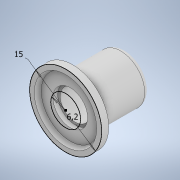
# Autodesk Inventor part: KnopfDuenn
Saved by Autodesk Inventor 2022.2 (Build 262287010, 287A)
## iProperties
Created: 2022-01-27
Part Number: KnopfDuenn
Material: Generisch
Document SubType Name: Modeling
Designer: hpcwoess
Density: 1 g/cm^3
Appearance: Vorgabe
Author: hpcwoess
Autodesk Inventor part; units mm, degrees
ref_plane "YZ Plane" through (0, 0, 0) normal (1, 0, 0) x (0, 1, 0)
ref_plane "XZ Plane" through (0, 0, 0) normal (0, 1, 0) x (-1, 0, 0)
ref_plane "XY Plane" through (0, 0, 0) normal (0, 0, 1) x (1, 0, 0)
sketch "Skizze1" plane through (0, 0, 0) normal (0, 0, 1) x (1, 0, 0)
  circle A0 centre (0, 0) radius 3.1
  circle A1 centre (0, 0) radius 7.5
  dimension "d0" = 6.2
  dimension "d1" = 15
  constraints: 2 centre point, 2 coincident
  measures "d0" diameter of A0
  measures "d1" diameter of A1
sketch "Skizze2" plane through (0, 0, 0) normal (1, 0, 0) x (0, 1, 0)
  line L0 (3.1, -2) -> (3.1, -11.5)
  line L1 (3.1, -11.5) -> (0, -11.5)
  line L2 (0, -11.5) -> (0, -12.5)
  line L3 (0, -12.5) -> (5, -12.5)
  line L4 (5, -12.5) -> (5, -2.5)
  line L5 (5, -2.5) -> (7.5, -1.5)
  line L6 (7.5, -1.5) -> (7.5, 0)
  line L7 (7.5, 0) -> (6.5, 0)
  line L8 (-10.5, 0) -> (10.5, 0) projected
  line L9 (0, -15) -> (0, 2.5) projected
  line L10 (3.6, -1) -> (3.6, -2)
  line L11 (3.6, -2) -> (3.1, -2)
  line L12 (3.6, -1) -> (6.05, -1)
  line L13 (6.05, -1) -> (6.5, 0)
  point P0 (0, 0)
  dimension "d7" = 11.5
  dimension "d8" = 1
  dimension "d10" = 1.5
  dimension "d11" = 3.1
  dimension "d12" = 7.5
  dimension "d13" = 1
  dimension "d16" = 3.6
  dimension "d17" = 2
  dimension "d18" = 5
  dimension "d19" = 1
  dimension "d20" = 6.5
  dimension "d21" = 0.45
  constraints: 24 end point, 7 perpendicular, 3 point on line, 1 horizontal, 1 parallel, 1 vertical
  measures "d7" distance from line of L1 point (0, 0)
  measures "d8" distance of L1.end L2.end
  measures "d10" distance of L5.end L6.end
  measures "d11" distance from line of point (0, 0) L0
  measures "d12" distance from line of point (0, 0) L6
  measures "d13" vertical distance of L5.end L4.end
  measures "d16" distance from line of L10 point (0, 0)
  measures "d17" distance from line of point (0, 0) L11
  measures "d18" distance from line of L4 point (0, 0)
  measures "d19" distance from line of point (0, 0) L12
  measures "d20" distance of L7.end point (0, 0)
  measures "d21" horizontal distance of L7.end L12.end
revolve "Umdrehung1" add sketch "Skizze2" angle 360 about axis through (0, 0, -10) along (0, 0, 1) contours L11 L10 L12 L13 L7 L6 L5 L4 L3 L2 L1 L0
fillet "Rundung2" radius 1 1 edges at (0, -5, -12.5)
